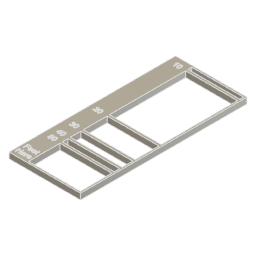
Range Finder - Human v2 (Autodesk Fusion 360 design; units mm, degrees)
Autodesk Fusion 360 part; units mm, degrees
sketch "Sketch1" plane through (0, 0, 0) normal (0, 1, 0) x (1, 0, 0)
  line L0 (38.1, 88.9) -> (-38.1, 88.9)
  line L1 (-38.1, 88.9) -> (-38.1, -88.9)
  line L2 (-38.1, -88.9) -> (38.1, -88.9)
  line L3 (38.1, -88.9) -> (38.1, 88.9)
  line L4 (-38.1, 88.9) -> (-35.56, 88.9) construction
  line L5 (38.1, -88.9) -> (36.3039, -87.1039)
  line L6 (38.1, -88.9) -> (40.64, -88.9) construction
  line L7 (-36.3039, 87.1039) -> (36.3039, 87.1039)
  line L8 (36.3039, 87.1039) -> (36.3039, -87.1039)
  line L9 (36.3039, -87.1039) -> (-19.05, -87.1039)
  line L10 (-38.1, 87.1039) -> (-19.05, 87.1039)
  line L11 (-19.05, 87.1039) -> (-19.05, -87.1039)
  dimension "d2" = 2.54
  dimension "d4" = 135
  dimension "d5" = 2.54
  dimension "d6" = 19.05
  constraint horizontal L0
  constraint vertical L1
  constraint horizontal L2
  constraint vertical L3
  constraint horizontal L4
  constraint horizontal L6
  constraint horizontal L7
  constraint vertical L8
  constraint horizontal L9
  constraint coincident L1 L10.start
  constraint coincident L7 L10.end
  constraint perpendicular L1 L10
  constraint coincident L9 L11.end
  constraint perpendicular L9 L11
  measures "d2" distance of L0.end L7.start
  measures "d4" angle of L5 L6
  measures "d5" distance of L2.end L5.end
  measures "d6" distance of L10.start L10.end
extrude "Extrude1" add sketch "Sketch1" along normal blind 6.35 contours L0 L1 L3 L5 L7 L8 L10 | L1 L2 L5 L7 L9 L10 L11
sketch "Sketch2" plane through (0, 6.35, 0) normal (0, 1, 0) x (-1, 0, 0)
  line L0 (19.05, -87.1039) -> (-36.3039, -87.1039)
  line L1 (-36.3039, -87.1039) -> (-36.3039, 87.1039)
  line L2 (-36.3039, 87.1039) -> (19.05, 87.1039)
  line L3 (19.05, 87.1039) -> (19.05, -87.1039)
  line L4 (-38.1, 88.9) -> (-38.1, -88.9)
  line L5 (-38.1, -88.9) -> (38.1, -88.9)
  line L6 (38.1, -88.9) -> (38.1, 88.9)
  line L7 (38.1, 88.9) -> (-38.1, 88.9)
  line L8 (19.05, -80.5361) -> (-36.3039, -80.5361)
  line L9 (-36.3039, -80.5361) -> (-36.3039, -83.0761)
  line L10 (-36.3039, -83.0761) -> (19.05, -83.0761)
  line L11 (19.05, -83.0761) -> (19.05, -80.5361)
  line L12 (19.05, 3.2839) -> (-36.3039, 3.2839)
  line L13 (-36.3039, 3.2839) -> (-36.3039, 0.7439)
  line L14 (-36.3039, 0.7439) -> (19.05, 0.7439)
  line L15 (19.05, 0.7439) -> (19.05, 3.2839)
  line L16 (19.05, 31.2239) -> (-36.3039, 31.2239)
  line L17 (-36.3039, 31.2239) -> (-36.3039, 28.6839)
  line L18 (-36.3039, 28.6839) -> (19.05, 28.6839)
  line L19 (19.05, 28.6839) -> (19.05, 31.2239)
  line L20 (19.05, 45.1939) -> (-36.3039, 45.1939)
  line L21 (-36.3039, 45.1939) -> (-36.3039, 42.6539)
  line L22 (-36.3039, 42.6539) -> (19.05, 42.6539)
  line L23 (19.05, 42.6539) -> (19.05, 45.1939)
  line L24 (19.05, 53.5759) -> (-36.3039, 53.5759)
  line L25 (-36.3039, 53.5759) -> (-36.3039, 51.0359)
  line L26 (-36.3039, 51.0359) -> (19.05, 51.0359)
  line L27 (19.05, 51.0359) -> (19.05, 53.5759)
  dimension "d9" = 167.64
  dimension "d10" = 2.54
  dimension "d11" = 83.82
  dimension "d12" = 2.54
  dimension "d13" = 55.88
  dimension "d14" = 2.54
  dimension "d15" = 41.91
  dimension "d16" = 2.54
  dimension "d17" = 33.528
  dimension "d18" = 2.54
  constraint horizontal L8
  constraint vertical L9
  constraint horizontal L10
  constraint vertical L11
  constraint coincident L1 L9.end
  constraint coincident L3 L12.start
  constraint horizontal L12
  constraint vertical L13
  constraint horizontal L14
  constraint vertical L15
  constraint coincident L1 L13.end
  constraint horizontal L16
  constraint vertical L17
  constraint horizontal L18
  constraint vertical L19
  constraint coincident L3 L20.start
  constraint horizontal L20
  constraint vertical L21
  constraint horizontal L22
  constraint vertical L23
  constraint coincident L1 L21.end
  constraint horizontal L24
  constraint vertical L25
  constraint horizontal L26
  constraint vertical L27
  constraint coincident L1 L25.end
  measures "d9" distance of L2.end L8.start
  measures "d10" distance of L8.start L10.end
  measures "d11" distance of L2.end L12.start
  measures "d12" distance of L12.start L14.end
  measures "d13" distance of L2.end L16.start
  measures "d14" distance of L16.start L18.end
  measures "d15" distance of L2.end L20.start
  measures "d16" distance of L20.start L22.end
  measures "d17" distance of L2.end L24.start
  measures "d18" distance of L24.start L26.end
extrude "Extrude2" add sketch "Sketch2" against normal blind 6.35 contours L1 L3 L8 L9 L10 L11 | L1 L3 L12 L13 L14 L15 | L1 L3 L16 L17 L18 L19 | L1 L3 L20 L21 L22 L23 | L1 L3 L24 L25 L26 L27
sketch "Sketch3" plane through (0, 6.35, 0) normal (0, 1, 0) x (-1, 0, 0)
  line L0 (-36.3039, 53.5759) -> (-36.3039, 87.1039)
  line L1 (-36.3039, 87.1039) -> (19.05, 87.1039)
  line L2 (19.05, 87.1039) -> (19.05, 53.5759)
  line L3 (19.05, 53.5759) -> (-36.3039, 53.5759)
  line L4 (-36.3039, -80.5361) -> (-36.3039, 0.7439)
  line L5 (-36.3039, 0.7439) -> (19.05, 0.7439)
  line L6 (19.05, 0.7439) -> (19.05, -80.5361)
  line L7 (19.05, -80.5361) -> (-36.3039, -80.5361)
  line L8 (-36.3039, 51.0359) -> (19.05, 51.0359)
  line L9 (19.05, 51.0359) -> (19.05, 45.1939)
  line L10 (19.05, 45.1939) -> (-36.3039, 45.1939)
  line L11 (-36.3039, 45.1939) -> (-36.3039, 51.0359)
  line L12 (-36.3039, 3.2839) -> (-36.3039, 28.6839)
  line L13 (-36.3039, 28.6839) -> (19.05, 28.6839)
  line L14 (19.05, 28.6839) -> (19.05, 3.2839)
  line L15 (19.05, 3.2839) -> (-36.3039, 3.2839)
  line L16 (-36.3039, 42.6539) -> (19.05, 42.6539)
  line L17 (19.05, 42.6539) -> (19.05, 31.2239)
  line L18 (19.05, 31.2239) -> (-36.3039, 31.2239)
  line L19 (-36.3039, 31.2239) -> (-36.3039, 42.6539)
  line L20 (-36.3039, -83.0761) -> (19.05, -83.0761)
  line L21 (19.05, -83.0761) -> (19.05, -87.1039)
  line L22 (19.05, -87.1039) -> (-36.3039, -87.1039)
  line L23 (-36.3039, -87.1039) -> (-36.3039, -83.0761)
  line L24 (-38.1, 88.9) -> (-38.1, -88.9)
  line L25 (-38.1, -88.9) -> (38.1, -88.9)
  line L26 (38.1, -88.9) -> (38.1, 88.9)
  line L27 (38.1, 88.9) -> (-38.1, 88.9)
  line L28 (34.5737, -73.8928) -> (21.5842, -73.6524) construction
  line L29 (21.5842, -73.6524) -> (21.3063, -88.6672) construction
  line L30 (21.3063, -88.6672) -> (34.2958, -88.9076) construction
  line L31 (34.2958, -88.9076) -> (34.5737, -73.8928) construction
  line L32 (35.56, 10.16) -> (22.86, 10.16) construction
  line L33 (22.86, 10.16) -> (22.86, -5.08) construction
  line L34 (22.86, -5.08) -> (35.56, -5.08) construction
  line L35 (35.56, -5.08) -> (35.56, 10.16) construction
  line L36 (34.6475, 35.3626) -> (21.9475, 35.3626) construction
  line L37 (21.9475, 35.3626) -> (21.9475, 22.6626) construction
  line L38 (21.9475, 22.6626) -> (34.6475, 22.6626) construction
  line L39 (34.6475, 22.6626) -> (34.6475, 35.3626) construction
  line L40 (35.56, 48.1149) -> (20.9866, 48.1149) construction
  line L41 (20.9866, 48.1149) -> (20.9866, 38.1) construction
  line L42 (20.9866, 38.1) -> (35.56, 38.1) construction
  line L43 (35.56, 38.1) -> (35.56, 48.1149) construction
  line L44 (33.9892, 57.3102) -> (22.1757, 57.3102) construction
  line L45 (22.1757, 57.3102) -> (22.1757, 47.3861) construction
  line L46 (22.1757, 47.3861) -> (33.9892, 47.3861) construction
  line L47 (33.9892, 47.3861) -> (33.9892, 57.3102) construction
  line L48 (36.83, 87.63) -> (20.32, 87.63) construction
  line L49 (20.32, 87.63) -> (20.32, 68.58) construction
  line L50 (20.32, 68.58) -> (36.83, 68.58) construction
  line L51 (36.83, 68.58) -> (36.83, 87.63) construction
  dimension "d21" = 5.08
  dimension "d22" = 0
  dimension "d23" = 5.08
  dimension "d24" = 0
  dimension "d25" = 5.08
  dimension "d26" = 0
  dimension "d27" = 5.08
  dimension "d28" = 0
  dimension "d29" = 5.08
  dimension "d30" = 0
  dimension "d31" = 5.08
  text T0 "10" font "Arial" height 5.08 align centre middle in box 12.9917 x 15.0173 at (34.5737, -73.8928) x (-0.999829, 0.018506) y (-0.018506, -0.999829) spacing 1
  text T1 "20" font "Arial" height 5.08 align centre middle in box 12.7 x 15.24 at (35.56, 10.16) x (-1, 0) y (0, -1) spacing 1
  text T2 "30" font "Arial" height 5.08 align centre middle in box 12.7 x 12.7 at (34.6475, 35.3626) x (-1, 0) y (0, -1) spacing 1
  text T3 "40" font "Arial" height 5.08 align centre middle in box 14.5734 x 10.0149 at (35.56, 48.1149) x (-1, 0) y (0, -1) spacing 1
  text T4 "50" font "Arial" height 5.08 align centre middle in box 11.8135 x 9.9241 at (33.9892, 57.3102) x (-1, 0) y (0, -1) spacing 1
  text T5 "Feet\nHere" font "Arial" height 5.08 align centre middle in box 16.51 x 19.05 at (36.83, 87.63) x (-1, 0) y (0, -1) spacing 1
extrude "Extrude3" cut sketch "Sketch3" against normal blind 1.27 text T0 T1 T2 T3 T4 T5
equation "d22 = '10'"
equation "d24 = '20'"
equation "d26 = '30'"
equation "d28 = '40'"
equation "d30 = '50'"
equation "d32 = 'Feet Here'"
